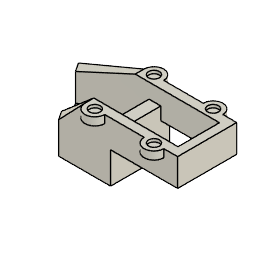
colour_detection_mechanism (Autodesk Fusion 360 archive; units mm, degrees)
design "Colour Sensor Holder"
part number: 2025-08-24-10-22-08-973
Autodesk Fusion 360 part; units mm, degrees
sketch "Base" plane through (0, 0, 0) normal (0, 0, 1) x (1, 0, 0)
  line L0 (0, 0) -> (46.334, 0)
  line L1 (46.334, 0) -> (46.334, 30)
  line L2 (46.334, 30) -> (0, 30)
  line L3 (0, 30) -> (0, 0)
  dimension "d2" = 46.334
  dimension "d3" = 30
  constraint horizontal L0
  constraint vertical L1
  constraint horizontal L2
  constraint vertical L3
  constraint coincident L0.start L3.end
  measures "d2" distance of L0.start L0.end
  measures "d3" distance of L0.end L1.end
extrude "Extrude1" add sketch "Base" along normal blind 4
sketch "Side Profile" plane through (0, 0, 0) normal (0, -1, 0) x (1, 0, 0)
  line L0 (0, 0) -> (46.334, 0)
  line L1 (46.334, 0) -> (46.334, 4)
  line L2 (46.334, 4) -> (0, 4)
  line L3 (0, 4) -> (0, 0)
  line L4 (46.334, 4) -> (46.334, 16)
  line L5 (46.334, 16) -> (80.334, 16)
  line L6 (80.334, 16) -> (80.334, 30)
  line L7 (80.334, 30) -> (0, 30)
  line L8 (0, 30) -> (0, 4)
  dimension "d6" = 12
  dimension "d7" = 34
  dimension "d8" = 14
  dimension "d11" = 46.334
  dimension "d52" = 80.334
  constraint coincident L1.end L2.start
  constraint perpendicular L2 L4
  constraint perpendicular L4 L5
  constraint perpendicular L5 L6
  constraint perpendicular L6 L7
  constraint coincident L2.end L3.start
  constraint perpendicular L2 L8
  measures "d6" distance of L1.end L4.end
  measures "d7" distance of L4.end L5.end
  measures "d8" distance of L5.end L6.end
  measures "d11" distance of L0.start L0.end
  measures "d52" distance of L6.end L7.end
extrude "Extrude2" add sketch "Side Profile" against normal blind 4.5 contours L2 L4 L5 L6 L7 L8
extrude "Extrude3" add sketch "Side Profile" against normal blind 4.5 from surface at -25.5 contours L2 L4 L5 L6 L7 L8
sketch "Front End" plane through (0, 0, 0) normal (0, -1, 0) x (1, 0, 0)
  line L0 (0, 0) -> (46.334, 0)
  line L1 (46.334, 0) -> (46.334, 16)
  line L2 (46.334, 16) -> (80.334, 16)
  line L3 (80.334, 16) -> (80.334, 30)
  line L4 (80.334, 30) -> (0, 30)
  line L5 (0, 30) -> (0, 0)
  line L6 (80.334, 30) -> (76.034, 30)
  line L7 (76.034, 30) -> (76.034, 16)
  line L8 (76.034, 16) -> (80.334, 16)
  line L9 (80.334, 16) -> (80.334, 30)
  dimension "d17" = 4.3
  constraint horizontal L6
  constraint vertical L7
  constraint horizontal L8
  constraint vertical L9
  constraint coincident L3.end L4.start
  constraint collinear L2 L8
  measures "d17" distance of L3.end L6.end
extrude "Extrude4" add sketch "Front End" against normal blind 30 contours L2 L3 L4 L6 L7 L8 L9
sketch "Middle End" plane through (0, 0, 0) normal (0, -1, 0) x (1, 0, 0)
  line L0 (80.334, 30) -> (0, 30)
  line L1 (0, 30) -> (0, 0)
  line L2 (0, 0) -> (46.334, 0)
  line L3 (46.334, 0) -> (46.334, 16)
  line L4 (46.334, 16) -> (80.334, 16)
  line L5 (80.334, 16) -> (80.334, 30)
  line L6 (46.334, 22.5) -> (40.334, 22.5)
  line L7 (40.334, 22.5) -> (40.334, 0)
  line L8 (40.334, 0) -> (46.334, 0)
  line L9 (46.334, 0) -> (46.334, 22.5)
  dimension "d20" = 7.5
  dimension "d21" = 6
  constraint horizontal L6
  constraint vertical L7
  constraint horizontal L8
  constraint vertical L9
  constraint collinear L3 L9
  constraint collinear L2 L8
  measures "d20" distance of L0 L6
  measures "d21" distance of L6.start L6.end
extrude "Extrude5" add sketch "Middle End" against normal blind 30 contours L2 L3 L6 L7 L8 L9
sketch "Lip" plane through (76.034, 0, 0) normal (-1, 0, 0) x (0, -1, 0)
  line L0 (-25.5, 30) -> (-25.5, 16)
  line L1 (-25.5, 16) -> (-4.5, 16)
  line L2 (-4.5, 16) -> (-4.5, 30)
  line L3 (-4.5, 30) -> (-25.5, 30)
  line L4 (-18, 25) -> (-12, 25)
  line L5 (-12, 25) -> (-12, 21)
  line L6 (-12, 21) -> (-18, 21)
  line L7 (-18, 21) -> (-18, 25)
  dimension "d24" = 5
  dimension "d25" = 6
  dimension "d26" = 4
  dimension "d27" = 7.5
  constraint horizontal L4
  constraint vertical L5
  constraint horizontal L6
  constraint vertical L7
  measures "d24" distance of L3 L4
  measures "d25" distance of L4.start L4.end
  measures "d26" distance of L4.start L6.end
  measures "d27" distance of L0 L7
extrude "Extrude6" add sketch "Lip" along normal blind 4 contours L4 L5 L6 L7
sketch "Magnet Holders" plane through (0, 0, 30) normal (0, 0, 1) x (-1, 0, 0)
  line L0 (-80.334, -30) -> (0, -30)
  line L1 (0, -30) -> (0, -25.5)
  line L2 (0, -25.5) -> (-76.034, -25.5)
  line L3 (-76.034, -25.5) -> (-76.034, -4.5)
  line L4 (-76.034, -4.5) -> (0, -4.5)
  line L5 (0, -4.5) -> (0, 0)
  line L6 (0, 0) -> (-80.334, 0)
  line L7 (-80.334, 0) -> (-80.334, -30)
  circle A0 centre (-68.334, -30) radius 5
  circle A1 centre (-38.334, -30) radius 5
  circle A2 centre (-38.334, 0) radius 5
  circle A3 centre (-68.334, 0) radius 5
  circle A4 centre (-38.334, 0) radius 2.75
  circle A5 centre (-68.334, 0) radius 2.75
  circle A6 centre (-38.334, -30) radius 2.75
  circle A7 centre (-68.334, -30) radius 2.75
  dimension "d33" = 10
  dimension "d34" = 10
  dimension "d35" = 10
  dimension "d36" = 10
  dimension "d37" = 12
  dimension "d38" = 12
  dimension "d43" = 5.5
  dimension "d44" = 5.5
  dimension "d45" = 5.5
  dimension "d46" = 5.5
  dimension "d50" = 42
  dimension "d51" = 42
  constraint coincident L0 A0.centre
  constraint coincident L0 A1.centre
  constraint coincident L6 A2.centre
  constraint coincident L6 A3.centre
  constraint concentric A2 A4
  constraint concentric A3 A5
  constraint concentric A1 A6
  constraint concentric A0 A7
  measures "d33" diameter of A0
  measures "d34" diameter of A1
  measures "d35" diameter of A2
  measures "d36" diameter of A3
  measures "d37" distance of L6.end A3.centre
  measures "d38" distance of L0.start A0.centre
  measures "d43" diameter of A4
  measures "d44" diameter of A5
  measures "d45" diameter of A6
  measures "d46" diameter of A7
  measures "d50" distance of L0.start A1.centre
  measures "d51" distance of L6.end A2.centre
extrude "Extrude8" add sketch "Magnet Holders" against normal blind 4 contours L0 A7 | L0 A0 A7 | L0 A1 A6 | L0 A6 | L6 A3 A5 | L6 A5 | L6 A2 A4 | L6 A4 picked at (-68.2655, -30.9141) picked at (-37.4674, -30.6679) picked at (-68.2655, 0.9141) picked at (-39.0365, 1.0303)
extrude "Extrude9" cut sketch "Magnet Holders" against normal blind 1.5 contours L0 A7 | L0 A7 | L0 A6 | L0 A6 | L6 A5 | L6 A5 | L6 A4 | L6 A4
sketch "Conduit Angle" plane through (0, 0, 30) normal (0, 0, 1) x (-1, 0, 0)
  circle A0 centre (-68.334, 0) radius 2.75
  circle A1 centre (-38.334, -30) radius 2.75
  circle A2 centre (-38.334, 0) radius 2.75
  circle A3 centre (-68.334, -30) radius 2.75
  line L0 (-33.334, -30) -> (0, -30)
  line L1 (0, -30) -> (0, -25.5)
  line L2 (0, -25.5) -> (-76.034, -25.5)
  line L3 (-76.034, -25.5) -> (-76.034, -4.5)
  line L4 (-76.034, -4.5) -> (0, -4.5)
  line L5 (0, -4.5) -> (0, 0)
  line L6 (0, 0) -> (-33.334, 0)
  arc A4 (-33.334, 0) -> (-43.334, 0) centre (-38.334, 0) ccw
  line L7 (-43.334, 0) -> (-63.334, 0)
  arc A5 (-63.334, 0) -> (-73.334, 0) centre (-68.334, 0) ccw
  line L8 (-73.334, 0) -> (-80.334, 0)
  line L9 (-80.334, 0) -> (-80.334, -30)
  line L10 (-80.334, -30) -> (-73.334, -30)
  arc A6 (-73.334, -30) -> (-63.334, -30) centre (-68.334, -30) ccw
  line L11 (-63.334, -30) -> (-43.334, -30)
  arc A7 (-43.334, -30) -> (-33.334, -30) centre (-38.334, -30) ccw
  line L12 (-40.334, -4.5) -> (-40.334, -25.5)
  line L13 (-40.334, -25.5) -> (0, -25.5)
  line L14 (0, -25.5) -> (0, -4.5)
  line L15 (0, -4.5) -> (-40.334, -4.5)
  line L16 (0, -30) -> (-19.932, 0)
  dimension "d53" = 33.6
  constraint coincident L0.end L1.start
  constraint coincident L6 L16.end
  measures "d53" angle of L14 L16
extrude "Extrude10" cut sketch "Conduit Angle" against normal blind 30 contours L1 L2 L13 L16 | L2 L4 L13 L14 L15 L16 | L4 L5 L6 L15 L16
sketch "Conduit Height" plane through (13.8279, 9.1873, 0) normal (-0.832921, -0.553392, 0) x (0.553392, -0.832921, 0)
  line L0 (-19.585, 4) -> (-19.585, 30)
  line L1 (-19.585, 30) -> (-24.9876, 30)
  line L2 (-24.9876, 30) -> (-24.9876, 0)
  line L3 (-24.9876, 0) -> (11.0302, 0)
  line L4 (11.0302, 0) -> (11.0302, 30)
  line L5 (11.0302, 30) -> (5.6275, 30)
  line L6 (5.6275, 30) -> (5.6275, 4)
  line L7 (5.6275, 4) -> (-19.585, 4)
  line L8 (-24.9876, 0) -> (11.0302, 0)
  line L9 (11.0302, 0) -> (11.0302, 16)
  line L10 (11.0302, 16) -> (-24.9876, 16)
  line L11 (-24.9876, 16) -> (-24.9876, 0)
  point P0 (5.6275, 16)
  point P1 (-19.585, 16)
  dimension "d56" = 16
  constraint horizontal L8
  constraint vertical L9
  constraint horizontal L10
  constraint vertical L11
  constraint coincident L4 L9.end
  constraint coincident L2.end L3.start
  constraint coincident L10 P0
  constraint coincident L6 P0
  constraint coincident L10 P1
  constraint coincident L0 P1
  measures "d56" distance of L8 L10
sketch "Colour Sensor Cover Shape" plane through (0, 0, 30) normal (0, 0, 1) x (-1, 0, 0)
  line L0 (0, -30) -> (-2.9898, -25.5)
  line L1 (-2.9898, -25.5) -> (-76.034, -25.5)
  line L2 (-76.034, -25.5) -> (-76.034, -4.5)
  line L3 (-76.034, -4.5) -> (-16.9422, -4.5)
  line L4 (-16.9422, -4.5) -> (-19.932, 0)
  line L5 (-19.932, 0) -> (-33.334, 0)
  arc A0 (-33.334, 0) -> (-43.334, 0) centre (-38.334, 0) ccw
  line L6 (-43.334, 0) -> (-63.334, 0)
  arc A1 (-63.334, 0) -> (-73.334, 0) centre (-68.334, 0) ccw
  line L7 (-73.334, 0) -> (-80.334, 0)
  line L8 (-80.334, 0) -> (-80.334, -30)
  line L9 (-80.334, -30) -> (-73.334, -30)
  arc A2 (-73.334, -30) -> (-63.334, -30) centre (-68.334, -30) ccw
  line L10 (-63.334, -30) -> (-43.334, -30)
  arc A3 (-43.334, -30) -> (-33.334, -30) centre (-38.334, -30) ccw
  line L11 (-33.334, -30) -> (0, -30)
  circle A4 centre (-68.334, 0) radius 2.75
  circle A5 centre (-38.334, -30) radius 2.75
  circle A6 centre (-38.334, 0) radius 2.75
  circle A7 centre (-68.334, -30) radius 2.75
  line L12 (-33.334, -30) -> (-33.334, 0)
  point P0 (-33.334, -25.5)
  point P1 (-33.334, -4.5)
  constraint coincident A3.end L11.start
  constraint coincident L5.end A0.start
  constraint coincident L1 P0
  constraint coincident L12 P0
  constraint coincident L3 P1
  constraint coincident L12 P1
sketch "Right Loft Outside Shape" plane through (0, 0, 0) normal (0, -1, 0) x (1, 0, 0)
  line L0 (19.932, 30) -> (19.932, 0)
  line L1 (19.932, 0) -> (46.334, 0)
  line L2 (46.334, 0) -> (46.334, 16)
  line L3 (46.334, 16) -> (80.334, 16)
  line L4 (80.334, 16) -> (80.334, 30)
  line L5 (80.334, 30) -> (73.334, 30)
  line L6 (73.334, 30) -> (73.334, 26)
  line L7 (73.334, 26) -> (63.334, 26)
  line L8 (63.334, 26) -> (63.334, 30)
  line L9 (63.334, 30) -> (43.334, 30)
  line L10 (43.334, 30) -> (43.334, 26)
  line L11 (43.334, 26) -> (33.334, 26)
  line L12 (33.334, 26) -> (33.334, 30)
  line L13 (33.334, 30) -> (19.932, 30)
  line L14 (33.334, 30) -> (19.932, 16)
  point P0 (33.334, 30)
  point P1 (19.932, 16)
  constraint coincident P0 L12.end
  constraint coincident P1 L14.end
sketch "Right Loft Inside Shape" plane through (0, 4.5, 0) normal (0, 1, 0) x (-1, 0, 0)
  line L0 (-16.9422, 4) -> (-16.9422, 30)
  line L1 (-16.9422, 30) -> (-76.034, 30)
  line L2 (-76.034, 30) -> (-76.034, 16)
  line L3 (-76.034, 16) -> (-46.334, 16)
  line L4 (-46.334, 16) -> (-46.334, 22.5)
  line L5 (-46.334, 22.5) -> (-40.334, 22.5)
  line L6 (-40.334, 22.5) -> (-40.334, 4)
  line L7 (-40.334, 4) -> (-16.9422, 4)
  line L8 (-33.334, 30) -> (-16.9422, 16)
  point P0 (-33.334, 30)
  point P1 (-16.9422, 16)
  constraint coincident P0 L8.start
  constraint coincident P1 L8.end
sketch "Left Loft Inside Shape" plane through (0, 25.5, 0) normal (0, -1, 0) x (1, 0, 0)
  line L0 (2.9898, 30) -> (2.9898, 4)
  line L1 (2.9898, 4) -> (40.334, 4)
  line L2 (40.334, 4) -> (40.334, 22.5)
  line L3 (40.334, 22.5) -> (46.334, 22.5)
  line L4 (46.334, 22.5) -> (46.334, 16)
  line L5 (46.334, 16) -> (76.034, 16)
  line L6 (76.034, 16) -> (76.034, 30)
  line L7 (76.034, 30) -> (2.9898, 30)
  line L8 (33.334, 30) -> (2.9898, 16)
  point P0 (33.334, 30)
  point P1 (2.9898, 16)
  constraint coincident P0 L8.start
  constraint coincident P1 L8.end
sketch "Left Loft Outside Shape" plane through (0, 30, 0) normal (0, 1, 0) x (-1, 0, 0)
  line L0 (-33.334, 30) -> (-33.334, 26)
  line L1 (-33.334, 26) -> (-43.334, 26)
  line L2 (-43.334, 26) -> (-43.334, 30)
  line L3 (-43.334, 30) -> (-63.334, 30)
  line L4 (-63.334, 30) -> (-63.334, 26)
  line L5 (-63.334, 26) -> (-73.334, 26)
  line L6 (-73.334, 26) -> (-73.334, 30)
  line L7 (-73.334, 30) -> (-80.334, 30)
  line L8 (-80.334, 30) -> (-80.334, 16)
  line L9 (-80.334, 16) -> (-46.334, 16)
  line L10 (-46.334, 16) -> (-46.334, 0)
  line L11 (-46.334, 0) -> (0, 0)
  line L12 (0, 0) -> (0, 30)
  line L13 (0, 30) -> (-33.334, 30)
  line L14 (-33.334, 30) -> (0, 16)
  point P0 (-33.334, 30)
  point P1 (0, 16)
  constraint coincident P0 L0.start
  constraint coincident P1 L14.end
loft "Loft1" cut profiles "Right Loft Outside Shape", "Right Loft Inside Shape" section 1 contours L0 L13 L14 section 2 contours L0 L1 L8
loft "Loft2" cut profiles "Left Loft Inside Shape", "Left Loft Outside Shape" section 1 contours L0 L7 L8 section 2 contours L12 L13 L14
chamfer "Chamfer2" distance 4 distance2 2 1 edges at (9.966, 15, 4) measured on face at (20.0887, 18.5, 4)
equation "base_plate_thickness = 4 mm" comment "Thickness of the Colour Detection Mechanism Platform's base plate."
equation "d4 = base_plate_thickness"
equation "d37 = 7 mm + 5 mm"
equation "d38 = 7 mm + 5 mm"
named bodies: "Colour Sensor Holder"

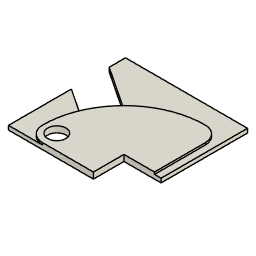
design "Colour Detection Mechanism Platform"
Autodesk Fusion 360 part; units mm, degrees
sketch "Colour Detection Mechanism Platform" plane through (0, 0, 0) normal (0, 0, 1) x (1, 0, 0)
  line L0 (0, 0) -> (120, 0)
  line L1 (120, 0) -> (120, 76)
  line L2 (120, 76) -> (0, 76)
  line L3 (0, 76) -> (0, 0)
  dimension "d169" = 120
  dimension "d170" = 76
  constraint horizontal L0
  constraint vertical L1
  constraint horizontal L2
  constraint vertical L3
  constraint coincident L0.start L3.end
  measures "d169" distance of L0.start L0.end
  measures "d170" distance of L0.start L2.end
extrude "Extrude42" add sketch "Colour Detection Mechanism Platform" along normal blind 4
sketch "Smartie Path" plane through (0, 0, 4) normal (0, 0, 1) x (-1, 0, 0)
  line L0 (0, -76) -> (0, 0)
  line L1 (0, 0) -> (-120, 0)
  line L2 (-120, 0) -> (-120, -76)
  line L3 (-120, -76) -> (0, -76)
  circle A0 centre (-98.5, 24) radius 80
  line L4 (-98.5, 24) -> (-113.5, 24)
  line L5 (-113.5, 24) -> (-113.5, -56)
  line L6 (-113.5, -56) -> (-98.5, -56)
  line L7 (-98.5, -56) -> (-98.5, 24)
  line L8 (-98.5, 24) -> (-18.5, 24)
  line L9 (-18.5, 24) -> (-18.5, 39)
  line L10 (-18.5, 39) -> (-98.5, 39)
  line L11 (-98.5, 39) -> (-98.5, 24)
  line L12 (-98.5, 24) -> (-113.5, 24)
  line L13 (-113.5, 24) -> (-113.5, 39)
  line L14 (-113.5, 39) -> (-98.5, 39)
  line L15 (-98.5, 39) -> (-98.5, 24)
  circle A1 centre (-32.5, 24) radius 9
  dimension "d173" = 160
  dimension "d174" = 24
  dimension "d175" = 21.5
  dimension "d176" = 15
  dimension "d177" = 15
  dimension "d178" = 80
  dimension "d179" = 80
  dimension "d184" = 18
  dimension "d185" = 14
  constraint horizontal L4
  constraint vertical L5
  constraint horizontal L6
  constraint vertical L7
  constraint coincident A0.centre L4.start
  constraint horizontal L8
  constraint vertical L9
  constraint horizontal L10
  constraint vertical L11
  constraint horizontal L12
  constraint vertical L13
  constraint horizontal L14
  constraint vertical L15
  constraint collinear L5 L13
  constraint collinear L10 L14
  constraint coincident L8 A1.centre
  measures "d173" diameter of A0
  measures "d174" distance of L1 A0.centre
  measures "d175" horizontal distance of L1.end A0.centre
  measures "d176" distance of L8.end L9.end
  measures "d177" distance of L5.end L6.end
  measures "d178" distance of L4.end L5.end
  measures "d179" distance of L9.end L10.end
  measures "d184" diameter of A1
  measures "d185" distance of L8.end A1.centre
extrude "Extrude43" add sketch "Smartie Path" along normal blind 2 contours L1 A0 L7 | L1 A0 L7 L8 A1 | L1 A0 L5 L7 | L1 L4 L5 L7 L12 | A0 L8 L10 L11 L15 A1 | L4 L11 L12 L13 L14 L15
fillet "Fillet2" radius 15 2 edges at (19.9188, -39, 5) (113.5, 54.5812, 5)
extrude "Extrude44" add 1 faces at (89.4665, -20.5529, 4) along direction (0, 0, -1) blind 4
sketch "Servo Hole" plane through (0, 0, 6) normal (0, 0, 1) x (-1, 0, 0)
  circle A0 centre (-32.5, 24) radius 9
  arc A1 (-113.5, -41) -> (-98.5, -56) centre (-98.5, -41) ccw
  arc A2 (-98.5, -56) -> (-18.5, 24) centre (-98.5, 24) ccw
  arc A3 (-18.5, 24) -> (-33.5, 39) centre (-33.5, 24) ccw
  line L0 (-33.5, 39) -> (-113.5, 39)
  line L1 (-113.5, 39) -> (-113.5, -41)
  line L2 (-113.5, 39) -> (-83.5, 39)
  line L3 (-83.5, 39) -> (-83.5, 9)
  line L4 (-83.5, 9) -> (-113.5, 9)
  line L5 (-113.5, 9) -> (-113.5, 39)
  dimension "d188" = 30
  dimension "d189" = 30
  constraint horizontal L2
  constraint vertical L3
  constraint horizontal L4
  constraint vertical L5
  constraint coincident L0.end L1.start
  measures "d188" distance of L3.end L4.end
  measures "d189" distance of L2.end L3.end
extrude "Extrude45" cut sketch "Servo Hole" against normal blind 6 contours L0 L1 L2 L3 L4 L5
sketch "Colour Sensor Holder Hole" plane through (0, 0, 4) normal (0, 0, 1) x (-1, 0, 0)
  line L0 (-120, 0) -> (-120, -76)
  line L1 (-120, -76) -> (0, -76)
  line L2 (0, -76) -> (0, 0)
  line L3 (-113.5, 0) -> (-120, 0)
  arc A0 (-98.5, -56) -> (-22.1849, 0) centre (-98.5, 24) ccw
  arc A1 (-113.5, -41) -> (-98.5, -56) centre (-98.5, -41) ccw
  line L4 (-113.5, -41) -> (-113.5, 0)
  line L5 (0, -59.401) -> (-38.732, -33.6675)
  line L6 (0, -23.4021) -> (-22.139, -8.693)
  line L7 (-38.732, -33.6675) -> (-22.139, -8.693)
  line L8 (0, -60.0013) -> (-39.4252, -33.8073)
  line L9 (-39.4252, -33.8073) -> (-22.2788, -7.9998)
  line L10 (-22.2788, -7.9998) -> (0, -22.8018)
  line L11 (0, 0) -> (-22.1849, 0)
  dimension "d249" = 56.4
  dimension "d250" = 59.401
  dimension "d254" = 56.4
  dimension "d255" = 8.693
  dimension "d256" = 22.139
  dimension "d257" = 23.4021
  dimension "d258" = 38.732
  dimension "d261" = 0.5
  dimension "d262" = 0.5
  dimension "d263" = 0.5
  constraint coincident L2 L5.start
  constraint coincident L2 L6.start
  constraint coincident L2 L8.start
  constraint coincident L2 L10.end
  constraint perpendicular L9 L10
  constraint parallel L5 L8
  constraint parallel L7 L9
  measures "d249" angle of L2 L5
  measures "d250" distance of L2.end L5.start
  measures "d254" angle of L2 L6
  measures "d255" distance of L3 L6.end
  measures "d256" horizontal distance of L2.end L6.end
  measures "d257" distance of L2.end L6.start
  measures "d258" horizontal distance of L5.start L5.end
  measures "d261" distance of L5 L8
  measures "d262" distance of L7 L9
extrude "Extrude58" cut sketch "Colour Sensor Holder Hole" against normal blind 4 contours L2 L5 L6 L7
extrude "Extrude59" cut sketch "Colour Sensor Holder Hole" against normal blind 4 contours L2 L5 L6 L7 L8 L9 L10
sketch "Platform Extension" plane through (0, 0, 4) normal (0, 0, 1) x (-1, 0, 0)
  line L0 (-22.2788, -7.9998) -> (0, -22.8018)
  line L1 (0, -22.8018) -> (0, 0)
  line L2 (0, 0) -> (-22.1849, 0)
  arc A0 (-98.5, -56) -> (-22.1849, 0) centre (-98.5, 24) ccw
  arc A1 (-113.5, -41) -> (-98.5, -56) centre (-98.5, -41) ccw
  line L3 (-113.5, -41) -> (-113.5, 0)
  line L4 (-120, 0) -> (-120, -76)
  line L5 (-120, -76) -> (0, -76)
  line L6 (0, -60.0013) -> (-39.4252, -33.8073)
  line L7 (-39.4252, -33.8073) -> (-22.2788, -7.9998)
  line L8 (-83.5, 9) -> (-113.5, 9)
  line L9 (-113.5, 9) -> (-113.5, -41)
  arc A2 (-113.5, -41) -> (-98.5, -56) centre (-98.5, -41) ccw
  arc A3 (-98.5, -56) -> (-18.5, 24) centre (-98.5, 24) ccw
  arc A4 (-18.5, 24) -> (-33.5, 39) centre (-33.5, 24) ccw
  line L10 (-33.5, 39) -> (-83.5, 39)
  line L11 (-83.5, 39) -> (-83.5, 9)
  circle A5 centre (-32.5, 24) radius 9
  line L12 (0, 0) -> (0, 39)
  line L13 (0, 39) -> (-33.5, 39)
  line L14 (-113.5, 0) -> (-120, 0)
  line L15 (0, -76) -> (0, -60.0013)
  line L16 (-113.5, 0) -> (-120, 0)
  line L17 (-120, 0) -> (-120, 9)
  line L18 (-120, 9) -> (-113.5, 9)
  line L19 (-113.5, 9) -> (-113.5, 0)
  constraint coincident L1.end L2.start
  constraint coincident A4.end L10.start
  constraint perpendicular L2 L12
  constraint perpendicular L12 L13
  constraint horizontal L16
  constraint vertical L17
  constraint horizontal L18
  constraint vertical L19
  constraint coincident L3.end L14.start
  constraint collinear L4 L17
  constraint collinear L8 L18
extrude "Extrude60" add sketch "Platform Extension" against normal blind 4 contours L2 A3 A4 L12 L13 | L9 L14 L16 L17 L18 L19
equation "d95 = 4 mm + 1.5 mm"
equation "d103 = -( 29 mm - 16 mm )"
named bodies: "Colour Detection Mechanism Platform"

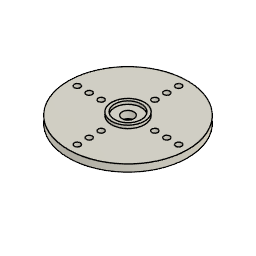
design "Savöx SH 0255 MG Micro Servo Horn"
description: Spur Gear; Module: 0.217; Num Teeth: 21; Pressure Angle: 20.0; Backlash: 0.00 mm
part number: 2026-07-12-11-53-48-100
Autodesk Fusion 360 part; units mm, degrees
sketch "Horn body" plane through (0, 0, 0) normal (0, 0, 1) x (1, 0, 0)
  circle A0 centre (0, 0) radius 10
  dimension "d1" = 20
  constraint coincident A0.centre origin
  measures "d1" diameter of A0
extrude "Extrude1" add sketch "Horn body" along normal blind 1.2 makes body 1
sketch "Connector" plane through (0, 0, 0) normal (0, 0, -1) x (1, 0, 0)
  circle A0 centre (0, 0) radius 10
  circle A1 centre (0, 0) radius 3.5
  dimension "d5" = 7
  constraint coincident A0.centre A1.centre
  measures "d5" diameter of A1
extrude "Extrude2" add sketch "Connector" along normal blind 3 contours A1 bodies 1
sketch "Screw hole" plane through (0, 0, 1.2) normal (0, 0, 1) x (-1, 0, 0)
  circle A0 centre (0, 0) radius 10
  circle A1 centre (0, 0) radius 2.75
  circle A2 centre (0, 0) radius 2.25
  circle A3 centre (0, 0) radius 1
  dimension "d8" = 5.5
  dimension "d9" = 4.5
  dimension "d10" = 2
  constraint coincident A0.centre A1.centre
  constraint concentric A2 A3
  measures "d8" diameter of A1
  measures "d9" diameter of A2
  measures "d10" diameter of A3
extrude "Extrude3" add sketch "Screw hole" along normal blind 0.5 contours A1 bodies 1
extrude "Extrude4" cut sketch "Screw hole" against normal blind 1.2 contours A3 bodies 1
sketch "Top small holes" plane through (0, 0, 1.2) normal (0, 0, 1) x (-1, 0, 0)
  circle A0 centre (0, 0) radius 10
  circle A1 centre (0, 0) radius 2.75
  circle A2 centre (0, -8.5) radius 0.5
  circle A3 centre (0, -6.5) radius 0.5
  circle A4 centre (0, -4.5) radius 0.5
  dimension "d15" = 1
  dimension "d16" = 1
  dimension "d17" = 1
  dimension "d19" = 8.5
  dimension "d20" = 6.5
  dimension "d21" = 4.5
  measures "d15" diameter of A2
  measures "d16" diameter of A3
  measures "d17" diameter of A4
  measures "d19" distance of A0.centre A2.centre
  measures "d20" distance of A0.centre A3.centre
  measures "d21" distance of A0.centre A4.centre
extrude "Extrude5" cut sketch "Top small holes" against normal blind 1.2 contours A2 | A3 | A4 bodies 1
pattern_circular "C-Pattern1" count 4 over 360 about axis through (0, 0, 1.75) along (0, 0, 1) of "Extrude5"
sketch "Base Circle" plane through (0, 0, 0) normal (0, 0, 1) x (1, 0, 0) in component "Savöx SH 0255 MG Micro Servo Gear"
  circle A0 centre (0, 0) radius 2.0274
extrude "Extrude1'" add sketch "Base Circle" along normal blind 3 separate body makes body 2 in component "Savöx SH 0255 MG Micro Servo Gear"
sketch "Gear Tooth" plane through (0, 0, 0) normal (0, 0, 1) x (1, 0, 0) in component "Savöx SH 0255 MG Micro Servo Gear"
  spline S0 degree 5 poles (2.1325, -0.1918) (2.1335, -0.1919) (2.1355, -0.1921) (2.1386, -0.1922) (2.1427, -0.1923) (2.1478, -0.1921) (2.1529, -0.1919) (2.1581, -0.1915) (2.1632, -0.191) (2.1683, -0.1906) (2.1735, -0.1901) (2.1787, -0.1895) (2.1838, -0.1889) (2.189, -0.1882) (2.1941, -0.1875) (2.1993, -0.1867) (2.2045, -0.1858) (2.2097, -0.1849) (2.2148, -0.1839) (2.22, -0.1829) (2.2252, -0.1818) (2.2304, -0.1807) (2.2356, -0.1796) (2.2407, -0.1784) (2.2459, -0.1772) (2.2511, -0.1759) (2.2563, -0.1746) (2.2615, -0.1732) (2.2667, -0.1718) (2.2719, -0.1703) (2.2771, -0.1689) (2.2823, -0.1674) (2.2875, -0.1658) (2.2927, -0.1642) (2.2979, -0.1626) (2.3031, -0.1609) (2.3083, -0.1592) (2.3134, -0.1575) (2.3186, -0.1557) (2.3238, -0.1539) (2.329, -0.152) (2.3342, -0.1502) (2.3394, -0.1482) (2.3446, -0.1463) (2.3498, -0.1443) (2.355, -0.1423) (2.3602, -0.1403) (2.3654, -0.1382) (2.3705, -0.1361) (2.3757, -0.1339) (2.3809, -0.1317) (2.3861, -0.1295) (2.3913, -0.1273) (2.3964, -0.125) (2.4016, -0.1227) (2.4068, -0.1204) (2.412, -0.118) (2.4171, -0.1156) (2.4223, -0.1132) (2.4275, -0.1107) (2.4326, -0.1082) (2.4378, -0.1057) (2.4429, -0.1032) (2.4481, -0.1006) (2.4532, -0.098) (2.4584, -0.0953) (2.4635, -0.0927) (2.4687, -0.09) (2.4738, -0.0872) (2.479, -0.0845) (2.4841, -0.0817) (2.4882, -0.0794) (2.4913, -0.0777) (2.4933, -0.0766) (2.4943, -0.076) knots 0 0 0 0 0 0 0.01428571 0.02857143 0.04285714 0.05714286 0.07142857 0.08571429 0.1 0.11428571 0.12857143 0.14285714 0.15714286 0.17142857 0.18571429 0.2 0.21428571 0.22857143 0.24285714 0.25714286 0.27142857 0.28571429 0.3 0.31428571 0.32857143 0.34285714 0.35714286 0.37142857 0.38571429 0.4 0.41428571 0.42857143 0.44285714 0.45714286 0.47142857 0.48571429 0.5 0.51428571 0.52857143 0.54285714 0.55714286 0.57142857 0.58571429 0.6 0.61428571 0.62857143 0.64285714 0.65714286 0.67142857 0.68571429 0.7 0.71428571 0.72857143 0.74285714 0.75714286 0.77142857 0.78571429 0.8 0.81428571 0.82857143 0.84285714 0.85714286 0.87142857 0.88571429 0.9 0.91428571 0.92857143 0.94285714 0.95714286 0.97142857 0.98571429 1 1 1 1 1 1
  spline S1 degree 5 poles (2.1325, 0.1918) (2.1335, 0.1919) (2.1355, 0.1921) (2.1386, 0.1922) (2.1427, 0.1923) (2.1478, 0.1921) (2.1529, 0.1919) (2.1581, 0.1915) (2.1632, 0.191) (2.1683, 0.1906) (2.1735, 0.1901) (2.1787, 0.1895) (2.1838, 0.1889) (2.189, 0.1882) (2.1941, 0.1875) (2.1993, 0.1867) (2.2045, 0.1858) (2.2097, 0.1849) (2.2148, 0.1839) (2.22, 0.1829) (2.2252, 0.1818) (2.2304, 0.1807) (2.2356, 0.1796) (2.2407, 0.1784) (2.2459, 0.1772) (2.2511, 0.1759) (2.2563, 0.1746) (2.2615, 0.1732) (2.2667, 0.1718) (2.2719, 0.1703) (2.2771, 0.1689) (2.2823, 0.1674) (2.2875, 0.1658) (2.2927, 0.1642) (2.2979, 0.1626) (2.3031, 0.1609) (2.3083, 0.1592) (2.3134, 0.1575) (2.3186, 0.1557) (2.3238, 0.1539) (2.329, 0.152) (2.3342, 0.1502) (2.3394, 0.1482) (2.3446, 0.1463) (2.3498, 0.1443) (2.355, 0.1423) (2.3602, 0.1403) (2.3654, 0.1382) (2.3705, 0.1361) (2.3757, 0.1339) (2.3809, 0.1317) (2.3861, 0.1295) (2.3913, 0.1273) (2.3964, 0.125) (2.4016, 0.1227) (2.4068, 0.1204) (2.412, 0.118) (2.4171, 0.1156) (2.4223, 0.1132) (2.4275, 0.1107) (2.4326, 0.1082) (2.4378, 0.1057) (2.4429, 0.1032) (2.4481, 0.1006) (2.4532, 0.098) (2.4584, 0.0953) (2.4635, 0.0927) (2.4687, 0.09) (2.4738, 0.0872) (2.479, 0.0845) (2.4841, 0.0817) (2.4882, 0.0794) (2.4913, 0.0777) (2.4933, 0.0766) (2.4943, 0.076) knots 0 0 0 0 0 0 0.01428571 0.02857143 0.04285714 0.05714286 0.07142857 0.08571429 0.1 0.11428571 0.12857143 0.14285714 0.15714286 0.17142857 0.18571429 0.2 0.21428571 0.22857143 0.24285714 0.25714286 0.27142857 0.28571429 0.3 0.31428571 0.32857143 0.34285714 0.35714286 0.37142857 0.38571429 0.4 0.41428571 0.42857143 0.44285714 0.45714286 0.47142857 0.48571429 0.5 0.51428571 0.52857143 0.54285714 0.55714286 0.57142857 0.58571429 0.6 0.61428571 0.62857143 0.64285714 0.65714286 0.67142857 0.68571429 0.7 0.71428571 0.72857143 0.74285714 0.75714286 0.77142857 0.78571429 0.8 0.81428571 0.82857143 0.84285714 0.85714286 0.87142857 0.88571429 0.9 0.91428571 0.92857143 0.94285714 0.95714286 0.97142857 0.98571429 1 1 1 1 1 1
  arc A0 (2.4943, -0.076) -> (2.4943, 0.076) centre (0, 0) ccw
  line L0 (2.0093, -0.1807) -> (2.1325, -0.1918)
  line L1 (2.0093, 0.1807) -> (2.1325, 0.1918)
  line L2 (2.0093, -0.1807) -> (2.0093, 0.1807)
  point P0 (2.1579, -0.1915)
  point P1 (2.1836, -0.1889)
  point P2 (2.2093, -0.1849)
  point P3 (2.2351, -0.1797)
  point P4 (2.261, -0.1733)
  point P5 (2.287, -0.1659)
  point P6 (2.3129, -0.1576)
  point P7 (2.3389, -0.1484)
  point P8 (2.3649, -0.1384)
  point P9 (2.3908, -0.1275)
  point P10 (2.4168, -0.1158)
  point P11 (2.4427, -0.1033)
  point P12 (2.4685, -0.09)
  point P13 (2.1579, 0.1915)
  point P14 (2.1836, 0.1889)
  point P15 (2.2093, 0.1849)
  point P16 (2.2351, 0.1797)
  point P17 (2.261, 0.1733)
  point P18 (2.287, 0.1659)
  point P19 (2.3129, 0.1576)
  point P20 (2.3389, 0.1484)
  point P21 (2.3649, 0.1384)
  point P22 (2.3908, 0.1275)
  point P23 (2.4168, 0.1158)
  point P24 (2.4427, 0.1033)
  point P25 (2.4685, 0.09)
extrude "Extrude2'" add sketch "Gear Tooth" along normal blind 3 bodies 2 in component "Savöx SH 0255 MG Micro Servo Gear"
fillet "Fillet1" radius 0.1 2 edges at (2.0193, -0.1816, 1.5) (2.0193, 0.1816, 1.5) on bodies 2 in component "Savöx SH 0255 MG Micro Servo Gear"
pattern_circular "C-Pattern1'" count 21 over 360 about axis through (0, 0, 0) along (0, 0, 1) of "Extrude2'", "Fillet1" in component "Savöx SH 0255 MG Micro Servo Gear"
sketch "Diametrial Pitch Circle" plane through (0, 0, 0) normal (0, 0, 1) x (1, 0, 0) in component "Savöx SH 0255 MG Micro Servo Gear"
  circle A0 centre (0, 0) radius 2.2785 construction
move_body "Move1" bodies 2 to x (1, 0, 0) y (0, 1, 0) z (0, 0, 1) at (0, 0, -3) in component "Savöx SH 0255 MG Micro Servo Gear"
combine "Combine1" operation cut target body 1 tool bodies 2 keep tools
component "Savöx SH 0255 MG Micro Servo Gear" placed x (1, 0, 0) y (0, 1, 0) z (0, 0, 1) at (0, 0, 0)
named bodies: "Savöx SH 0255 MG Micro Servo Horn", "Savöx SH 0255 MG Micro Servo Gear"

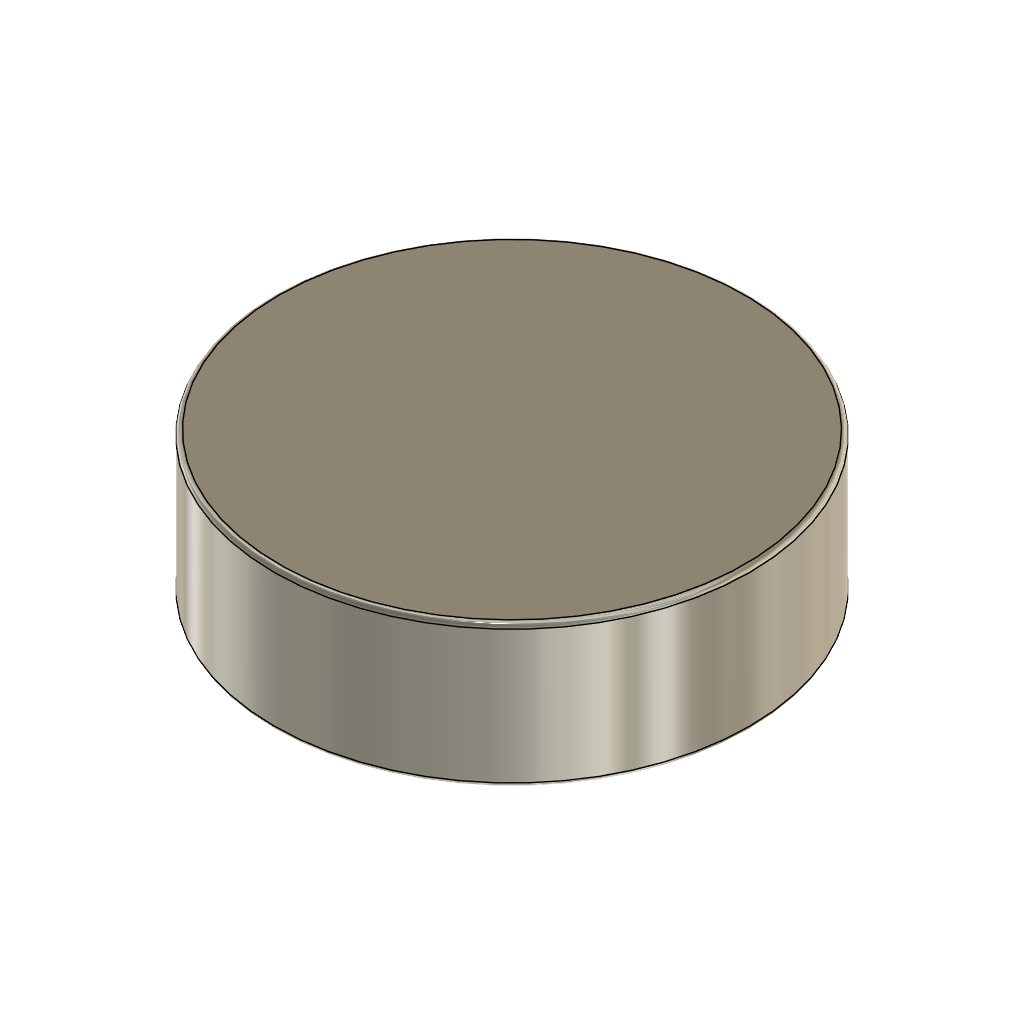
design "5 mm x 1.5 mm Neodymium Disc Magnet"
Autodesk Fusion 360 part; units mm, degrees
sketch "5 mm x 1.5 mm neodymium disc magnet" plane through (0, 0, 0) normal (0, 0, 1) x (1, 0, 0)
  circle A0 centre (0, 0) radius 2.5
  dimension "d1" = 5
  constraint coincident A0.centre origin
  measures "d1" diameter of A0
extrude "Extrude1" add sketch "5 mm x 1.5 mm neodymium disc magnet" along normal blind 1.5
fillet "Fillet1" radius 0.05 2 edges at (-2.3308, -0.904, 1.5) (-2.3308, -0.904, 0)
named bodies: "5 mm x 1.5 mm Neodymium Disc Magnet"

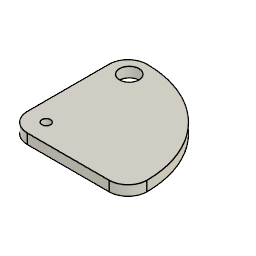
design "Smartie Arm"
Autodesk Fusion 360 part; units mm, degrees
sketch "Smartie arm" plane through (0, 0, 0) normal (0, 0, 1) x (1, 0, 0)
  line L0 (0, 0) -> (95, 0)
  line L1 (95, 0) -> (95, 95)
  line L2 (95, 95) -> (0, 95)
  line L3 (0, 95) -> (0, 0)
  dimension "d6" = 95
  dimension "d15" = 95
  constraint horizontal L0
  constraint vertical L1
  constraint horizontal L2
  constraint vertical L3
  constraint coincident L0.start L3.end
  measures "d6" distance of L1.end L2.end
  measures "d15" distance of L0.end L1.end
extrude "Extrude1" add sketch "Smartie arm" along normal blind 8
sketch "Smartie hole" plane through (0, 0, 8) normal (0, 0, 1) x (-1, 0, 0)
  line L0 (0, -95) -> (0, 0)
  line L1 (0, 0) -> (-95, 0)
  line L2 (-95, 0) -> (-95, -95)
  line L3 (-95, -95) -> (0, -95)
  circle A0 centre (-15, -81) radius 7.75
  dimension "d5" = 15.5
  dimension "d8" = 15
  dimension "d9" = 80
  dimension "d14" = 14
  measures "d5" diameter of A0
  measures "d8" distance of L0 A0.centre
  measures "d9" distance of L2 A0.centre
  measures "d14" distance of L3 A0.centre
extrude "Extrude2" cut sketch "Smartie hole" against normal blind 8 contours A0
fillet "Fillet1" radius 15 2 edges at (95, 95, 4) (0, 95, 4)
fillet "Fillet2" radius 15 2 edges at (0, 0, 4) (95, 0, 4)
sketch "Smartie arm arc" plane through (0, 0, 8) normal (0, 0, 1) x (-1, 0, 0)
  arc A0 (-80, 0) -> (-95, -15) centre (-80, -15) ccw
  line L0 (-95, -15) -> (-95, -80)
  arc A1 (-95, -80) -> (-80, -95) centre (-80, -80) ccw
  line L1 (-80, -95) -> (-15, -95)
  arc A2 (-15, -95) -> (0, -80) centre (-15, -80) ccw
  line L2 (0, -80) -> (0, -15)
  arc A3 (0, -15) -> (-15, 0) centre (-15, -15) ccw
  line L3 (-15, 0) -> (-80, 0)
  circle A4 centre (-15, -81) radius 7.75
  circle A5 centre (-15, -15) radius 80
  dimension "d16" = 15
  dimension "d17" = 15
  dimension "d18" = 160
  measures "d16" horizontal distance of L2.end A3.centre
  measures "d17" distance of L3 A3.centre
  measures "d18" diameter of A5
extrude "Extrude3" cut sketch "Smartie arm arc" against normal blind 8 contours L0 A1 L1 A5
sketch "Servo horn hole" plane through (0, 0, 0) normal (0, 0, -1) x (1, 0, 0)
  arc A0 (15, -95) -> (95, -15) centre (15, -15) ccw
  arc A1 (95, -15) -> (80, 0) centre (80, -15) ccw
  line L0 (80, 0) -> (15, 0)
  arc A2 (15, 0) -> (0, -15) centre (15, -15) ccw
  line L1 (0, -15) -> (0, -80)
  arc A3 (0, -80) -> (15, -95) centre (15, -80) ccw
  circle A4 centre (15, -81) radius 7.75
  circle A5 centre (15, -15) radius 10.25
  circle A6 centre (15, -15) radius 3.5
  dimension "d21" = 20.5
  dimension "d24" = 7
  constraint concentric A0 A5
  constraint concentric A5 A6
  measures "d21" diameter of A5
  measures "d24" diameter of A6
extrude "Extrude4" cut sketch "Servo horn hole" against normal blind 1.2 contours A5 | A6
extrude "Extrude5" cut sketch "Servo horn hole" against normal blind 8 contours A6
equation "d14 = 16 mm - 2 mm"
named bodies: "Smartie arm"

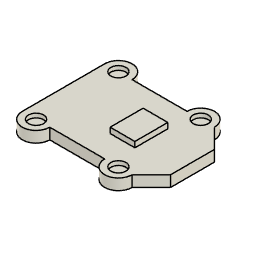
design "Colour Sensor Cover"
part number: 2025-08-25-11-06-01-160
Autodesk Fusion 360 part; units mm, degrees
sketch "Colour Sensor Cover" plane through (0, 0, 0) normal (0, 0, 1) x (1, 0, 0)
  line L0 (0, 0) -> (47, 0)
  line L1 (47, 0) -> (47, 30)
  line L2 (47, 30) -> (0, 30)
  line L3 (0, 30) -> (0, 0)
  circle A0 centre (5, 30) radius 5
  circle A1 centre (35, 30) radius 5
  circle A2 centre (5, 0) radius 5
  circle A3 centre (35, 0) radius 5
  dimension "d1" = 47
  dimension "d2" = 30
  dimension "d3" = 10
  dimension "d4" = 10
  dimension "d5" = 10
  dimension "d6" = 10
  dimension "d7" = 5
  dimension "d8" = 5
  dimension "d9" = 12
  dimension "d10" = 12
  constraint horizontal L0
  constraint vertical L1
  constraint horizontal L2
  constraint vertical L3
  constraint coincident L0.start L3.end
  constraint coincident L2 A0.centre
  constraint coincident L2 A1.centre
  constraint coincident L0 A2.centre
  constraint coincident L0 A3.centre
  measures "d1" distance of L0.start L0.end
  measures "d2" distance of L0.end L1.end
  measures "d3" diameter of A0
  measures "d4" diameter of A1
  measures "d5" diameter of A2
  measures "d6" diameter of A3
  measures "d7" distance of L2.end A0.centre
  measures "d8" distance of L0.start A2.centre
  measures "d9" distance of L1.end A1.centre
  measures "d10" distance of L0.end A3.centre
extrude "Extrude1" add sketch "Colour Sensor Cover" along normal blind 4
chamfer "Chamfer1" distance 7 angle 45 2 edges at (47, 0, 2) (47, 30, 2)
sketch "Magnet Holes" plane through (0, 0, 4) normal (0, 0, 1) x (-1, 0, 0)
  line L0 (-47, -23) -> (-40, -30)
  arc A0 (-40, -30) -> (-30, -30) centre (-35, -30) ccw
  line L1 (-30, -30) -> (-10, -30)
  arc A1 (-10, -30) -> (0, -30) centre (-5, -30) ccw
  line L2 (0, -30) -> (0, 0)
  arc A2 (0, 0) -> (-10, 0) centre (-5, 0) ccw
  line L3 (-10, 0) -> (-30, 0)
  arc A3 (-30, 0) -> (-40, 0) centre (-35, 0) ccw
  line L4 (-40, 0) -> (-47, -7)
  line L5 (-47, -7) -> (-47, -23)
  circle A4 centre (-5, -30) radius 2.75
  circle A5 centre (-35, -30) radius 2.75
  circle A6 centre (-5, 0) radius 2.75
  circle A7 centre (-35, 0) radius 2.75
  dimension "d14" = 5.5
  dimension "d15" = 5.5
  dimension "d16" = 5.5
  dimension "d17" = 5.5
  constraint concentric A1 A4
  constraint concentric A0 A5
  constraint concentric A2 A6
  constraint concentric A3 A7
  measures "d14" diameter of A4
  measures "d15" diameter of A5
  measures "d16" diameter of A6
  measures "d17" diameter of A7
extrude "Extrude2" cut sketch "Magnet Holes" against normal blind 1.5 contours A4 | A5 | A6 | A7
sketch "Colour Sensor Support" plane through (0, 0, 4) normal (0, 0, 1) x (-1, 0, 0)
  circle A0 centre (-5, -30) radius 2.75
  circle A1 centre (-35, -30) radius 2.75
  circle A2 centre (-5, 0) radius 2.75
  circle A3 centre (-35, 0) radius 2.75
  line L0 (-47, -23) -> (-40, -30)
  arc A4 (-40, -30) -> (-30, -30) centre (-35, -30) ccw
  line L1 (-30, -30) -> (-10, -30)
  arc A5 (-10, -30) -> (0, -30) centre (-5, -30) ccw
  line L2 (0, -30) -> (0, 0)
  arc A6 (0, 0) -> (-10, 0) centre (-5, 0) ccw
  line L3 (-10, 0) -> (-30, 0)
  arc A7 (-30, 0) -> (-40, 0) centre (-35, 0) ccw
  line L4 (-40, 0) -> (-47, -7)
  line L5 (-47, -7) -> (-47, -23)
  line L6 (-23, -21) -> (-32, -21)
  line L7 (-32, -21) -> (-32, -9)
  line L8 (-32, -9) -> (-23, -9)
  line L9 (-23, -9) -> (-23, -21)
  dimension "d20" = 9
  dimension "d21" = 9
  dimension "d22" = 15
  dimension "d23" = 9
  dimension "d24" = 12
  constraint horizontal L6
  constraint vertical L7
  constraint horizontal L8
  constraint vertical L9
  measures "d20" distance of L1 L6
  measures "d21" distance of L3 L8
  measures "d22" distance of L5 L7
  measures "d23" distance of L6.start L6.end
  measures "d24" distance of L6.end L7.end
extrude "Extrude3" add sketch "Colour Sensor Support" along normal blind 2 contours L6 L7 L8 L9
equation "d9 = 7 mm + 5 mm"
equation "d10 = 7 mm + 5 mm"
named bodies: "Colour Sensor Cover"

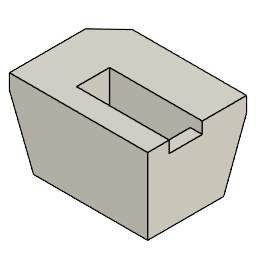
design "Colour Sensor Servo Seat"
part number: 2025-09-25-10-48-16-577
Autodesk Fusion 360 part; units mm, degrees
sketch "Colour Sensor Servo Seat Outline" plane through (0, 0, 0) normal (0, 0, 1) x (1, 0, 0)
  line L0 (0, 0) -> (54.5, 0)
  line L1 (54.5, 0) -> (54.5, 39)
  line L2 (54.5, 39) -> (0, 39)
  line L3 (0, 39) -> (0, 0)
  dimension "d1" = 39
  dimension "d2" = 54.5
  constraint horizontal L0
  constraint vertical L1
  constraint horizontal L2
  constraint vertical L3
  constraint coincident L0.start L3.end
  measures "d1" distance of L0.end L1.end
  measures "d2" distance of L0.start L0.end
extrude "Extrude1" add sketch "Colour Sensor Servo Seat Outline" along normal blind 30
sketch "Colour Sensor Servo Hole" plane through (0, 0, 30) normal (0, 0, 1) x (-1, 0, 0)
  line L0 (0, -39) -> (0, 0)
  line L1 (0, 0) -> (-54.5, 0)
  line L2 (-54.5, 0) -> (-54.5, -39)
  line L3 (-54.5, -39) -> (0, -39)
  line L4 (-54.5, -8.5) -> (-18, -8.5)
  line L5 (-18, -8.5) -> (-18, -21.5)
  line L6 (-18, -21.5) -> (-54.5, -21.5)
  line L7 (-54.5, -21.5) -> (-54.5, -8.5)
  line L8 (-54.5, 0) -> (-18, 0)
  line L9 (-18, 0) -> (-18, -30)
  line L10 (-18, -30) -> (-54.5, -30)
  line L11 (-54.5, -30) -> (-54.5, 0)
  line L12 (-54.5, -21.5) -> (-49.8, -21.5)
  line L13 (-49.8, -21.5) -> (-49.8, -8.5)
  line L14 (-49.8, -8.5) -> (-54.5, -8.5)
  line L15 (-54.5, -8.5) -> (-54.5, -21.5)
  point P0 (-54.5, -21.5)
  point P1 (-54.5, -30)
  dimension "d6" = 13
  dimension "d8" = 36.5
  dimension "d9" = 30
  dimension "d10" = 8.5
  dimension "d11" = 8.5
  dimension "d12" = 4.7
  constraint horizontal L4
  constraint vertical L5
  constraint horizontal L6
  constraint vertical L7
  constraint coincident L2 L4.start
  constraint horizontal L8
  constraint vertical L9
  constraint horizontal L10
  constraint vertical L11
  constraint coincident L1.end L2.start
  constraint collinear L5 L9
  constraint coincident P0 L6.end
  constraint coincident P1 L10.end
  constraint horizontal L12
  constraint vertical L13
  constraint horizontal L14
  constraint vertical L15
  constraint coincident L4 L13.end
  measures "d6" distance of L4.start P0
  measures "d8" distance of L4.start L4.end
  measures "d9" distance of L1.end P1
  measures "d10" distance of L6 L10
  measures "d11" distance of L4 L8
  measures "d12" distance of L11 L13
extrude "Extrude2" cut sketch "Colour Sensor Servo Hole" against normal blind 4.58 contours L2 L4 L6 L7 L11 L12 L13 L14 L15
extrude "Extrude3" cut sketch "Colour Sensor Servo Hole" against normal blind 25.4 contours L4 L5 L6 L9 L13
chamfer "Chamfer1" distance 24 distance2 9 1 edges at (27.25, 39, 0) measured on face at (36.3333, 39, 20)
sketch "Front Ribs" plane through (0, 39, 0) normal (0, 1, 0) x (-1, 0, 0)
  line L0 (-54.5, 24) -> (0, 24)
  line L1 (0, 24) -> (0, 30)
  line L2 (0, 30) -> (-54.5, 30)
  line L3 (-54.5, 30) -> (-54.5, 24)
  line L4 (0, 0) -> (0, 24)
  line L5 (0, 24) -> (-54.5, 24)
  line L6 (-54.5, 24) -> (-54.5, 0)
  line L7 (-54.5, 0) -> (0, 0)
  line L8 (-46, 24) -> (-18, 24)
  line L9 (-18, 24) -> (-18, 0)
  line L10 (-18, 0) -> (-46, 0)
  line L11 (-46, 0) -> (-46, 24)
  line L12 (-18, 24) -> (-9.5, 24)
  line L13 (-9.5, 24) -> (-9.5, 0)
  line L14 (-9.5, 0) -> (-18, 0)
  line L15 (-18, 0) -> (-18, 24)
  dimension "d26" = 8.5
  dimension "d31" = 8.5
  dimension "d39" = 9.5
  constraint horizontal L8
  constraint vertical L9
  constraint horizontal L10
  constraint vertical L11
  constraint coincident L7 L9.end
  constraint coincident L0 L8.start
  constraint horizontal L12
  constraint vertical L13
  constraint horizontal L14
  constraint vertical L15
  constraint coincident L7 L13.end
  measures "d26" distance of L6 L11
  measures "d31" distance of L13 L15
  measures "d39" distance of L4 L13
extrude "Extrude4" cut sketch "Front Ribs" against normal blind 9 contours L0 L5 L7 L8 L9 L10 L11 L15 | L0 L4 L5 L7 L13
chamfer "Chamfer2" distance 24 distance2 9.5 1 edges at (0, 15, 0) measured on face at (0, 10, 18)
sketch "Side Ribs" plane through (0, 0, 0) normal (-1, 0, 0) x (0, -1, 0)
  line L0 (-30, 24) -> (0, 24)
  line L1 (0, 24) -> (0, 30)
  line L2 (0, 30) -> (-39, 30)
  line L3 (-39, 30) -> (-39, 24)
  line L4 (-39, 24) -> (-30, 24)
  line L5 (0, 0) -> (0, 24)
  line L6 (0, 24) -> (-30, 24)
  line L7 (-30, 24) -> (-30, 0)
  line L8 (-30, 0) -> (0, 0)
  line L9 (-21.5, 24) -> (-8.5, 24)
  line L10 (-8.5, 24) -> (-8.5, 0)
  line L11 (-8.5, 0) -> (-21.5, 0)
  line L12 (-21.5, 0) -> (-21.5, 24)
  dimension "d33" = 8.5
  dimension "d34" = 8.5
  constraint horizontal L9
  constraint vertical L10
  constraint horizontal L11
  constraint vertical L12
  constraint coincident L8 L10.end
  constraint coincident L0 L9.start
  measures "d33" distance of L7 L12
  measures "d34" distance of L5 L10
extrude "Extrude6" cut sketch "Side Ribs" against normal blind 9.5 contours L0 L6 L8 L9 L10 L11 L12
chamfer "Chamfer3" distance 9.5 distance2 9 1 edges at (0, 39, 27) measured on face at (24.1667, 39, 28)
sketch "Servo Cable Hole" plane through (9.5, 0, 0) normal (-1, 0, 0) x (0, -1, 0)
  line L0 (-21.5, 0) -> (-8.5, 0)
  line L1 (-8.5, 0) -> (-8.5, 24)
  line L2 (-8.5, 24) -> (-21.5, 24)
  line L3 (-21.5, 24) -> (-21.5, 0)
  line L4 (-21.5, 0) -> (-21.5, 24)
  line L5 (-21.5, 24) -> (-30, 24)
  line L6 (-30, 24) -> (-30, 0)
  line L7 (-30, 0) -> (-21.5, 0)
  line L8 (-8.5, 24) -> (-8.5, 0)
  line L9 (-8.5, 0) -> (0, 0)
  line L10 (0, 0) -> (0, 24)
  line L11 (0, 24) -> (-8.5, 24)
  line L12 (-21.5, 14.6) -> (-8.5, 14.6)
  line L13 (-8.5, 14.6) -> (-8.5, 4.6)
  line L14 (-8.5, 4.6) -> (-21.5, 4.6)
  line L15 (-21.5, 4.6) -> (-21.5, 14.6)
  dimension "d40" = 10
  dimension "d41" = 4.6
  constraint horizontal L12
  constraint vertical L13
  constraint horizontal L14
  constraint vertical L15
  constraint coincident L4 L12.start
  measures "d40" distance of L12.start L14.end
  measures "d41" distance of L0 L14
extrude "Extrude7" cut sketch "Servo Cable Hole" against normal blind 8.5 contours L1 L3 L4 L8 L12 L13 L14 L15
equation "d2 = servo_seat_width"
equation "d3 = servo_seat_height"
equation "servo_seat_height = 30 mm" comment "The height of the Colour Sensor Servo Seat component."
equation "d6 = servo_hole_width"
equation "servo_hole_width = 13 mm" comment "The width of the hole for the Colour Sensor Servo to sit in."
equation "d10 = ( 30 mm - servo_hole_width ) / 2"
equation "d13 = -servo_arm_support_depth"
equation "servo_arm_support_depth = 5 mm - 0.42 mm" comment "The depth to extrude to create the arm support for the Colour Sensor Servo."
equation "servo_hole_depth = 25.82 mm - 0.42 mm" comment "The depth to extrude to create the hole for the Colour Sensor Servo to sit in."
equation "d17 = -servo_hole_depth"
equation "d19 = servo_seat_height - top_support_thickness"
equation "d20 = 17.50 mm - 8.50 mm"
equation "top_support_thickness = 6 mm" comment "The thickness of the top supports that will go underneath the Colour Detection Mechanism Platform."
equation "d22 = -( 17.50 mm - 8.50 mm )"
equation "rib_thickness = 8.5 mm" comment "The thickness of the support ribs."
equation "d26 = rib_thickness"
equation "d27 = servo_seat_height - top_support_thickness"
equation "d28 = servo_seat_width - 36.50 mm - 8.5 mm"
equation "d31 = rib_thickness"
equation "servo_seat_width = 36.50 mm + 18 mm" comment "The width of the Colour Sensor Servo Seat component."
equation "d33 = rib_thickness"
equation "d34 = rib_thickness"
equation "d35 = -( servo_seat_width - 36.50 mm - 8.5 mm )"
equation "d37 = ( servo_seat_width - 36.50 mm - 8.5 mm )"
equation "d39 = ( servo_seat_width - 36.50 mm - 8.5 mm )"
equation "d41 = servo_seat_height - servo_hole_depth"
equation "d42 = -rib_thickness"
named bodies: "Colour Sensor Servo Seat"
